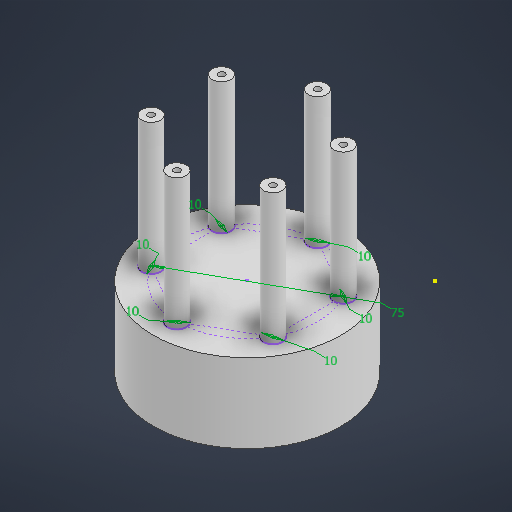
# Autodesk Inventor part: Pieza1
Saved by Autodesk Inventor 2026.1 (Build 301233000, 233)
## iProperties
Created: 2025-09-15
Part Number: Pieza1
Material: Genérico
Document SubType Name: Modeling
Designer: Usuario
Density: 1 g/cm^3
Appearance: Valor por defecto
Author: Usuario
Autodesk Inventor part; units mm, degrees
ref_plane "YZ Plane" through (0, 0, 0) normal (1, 0, 0) x (0, 1, 0)
ref_plane "XZ Plane" through (0, 0, 0) normal (0, 1, 0) x (-1, 0, 0)
ref_plane "XY Plane" through (0, 0, 0) normal (0, 0, 1) x (1, 0, 0)
sketch "Boceto1" plane through (0, 0, 0) normal (0, 1, 0) x (-1, 0, 0)
  line L0 (0, 0) -> (100, 0) construction
  line L1 (100, 0) -> (100, 100) construction
  line L2 (100, 100) -> (0, 100) construction
  line L3 (0, 100) -> (0, 0) construction
  line L4 (0, 100) -> (100, 0) construction
  line L5 (100, 100) -> (0, 0) construction
  circle A0 centre (50, 50) radius 50
  dimension "d2" = 100
  constraints: 12 end point, 2 parallel, 1 centre point, 1 horizontal, 1 midpoint, 1 perpendicular
  measures "d2" diameter of A0
extrude "Extrusión1" add sketch "Boceto1" along normal blind 35
sketch "Boceto2" plane through (-50, 35, 50) normal (0, 1, 0) x (1, 0, 0)
  circle A0 centre (0, 0) radius 37.5 construction
  line L0 (0, 37.5) -> (32.476, 18.75) construction
  line L1 (32.476, 18.75) -> (32.476, -18.75) construction
  line L2 (32.476, -18.75) -> (0, -37.5) construction
  line L3 (0, -37.5) -> (-32.476, -18.75) construction
  line L4 (-32.476, -18.75) -> (-32.476, 18.75) construction
  line L5 (-32.476, 18.75) -> (0, 37.5) construction
  circle A1 centre (0, 37.5) radius 5
  circle A2 centre (32.476, 18.75) radius 5
  circle A3 centre (32.476, -18.75) radius 5
  circle A4 centre (0, -37.5) radius 5
  circle A5 centre (-32.476, -18.75) radius 5
  circle A6 centre (-32.476, 18.75) radius 5
  point P0 (50, 50)
  dimension "d5" = 75
  dimension "d6" = 10
  dimension "d7" = 10
  dimension "d8" = 10
  dimension "d9" = 10
  dimension "d10" = 10
  dimension "d11" = 10
  constraints: 12 end point, 7 coincident, 6 centre point, 1 vertical alignment, 15 other
  measures "d6" diameter of A1
  measures "d7" diameter of A2
  measures "d8" diameter of A3
  measures "d9" diameter of A4
  measures "d10" diameter of A5
  measures "d11" diameter of A6
extrude "Extrusión2" add sketch "Boceto2" along normal blind 70
sketch "Boceto3" plane through (-82.476, 105, 68.75) normal (0, 1, 0) x (1, 0, 0)
  circle A0 centre (32.5355, 18.7491) radius 37.5 construction
  circle A1 centre (32.5355, -18.7509) radius 1.75
  circle A2 centre (65.012, 0) radius 1.75
  circle A3 centre (65.012, 37.4981) radius 1.75
  circle A4 centre (32.5355, 56.2491) radius 1.75
  circle A5 centre (0.059, 37.4981) radius 1.75
  circle A6 centre (0, 0) radius 5 projected
  circle A7 centre (0, 0) radius 1.75
  point P0 (82.476, 68.75)
  dimension "d15" = 3.5
  dimension "d16" = 3.5
  dimension "d17" = 3.5
  dimension "d18" = 3.5
  dimension "d19" = 3.5
  dimension "d20" = 3.5
  constraints: 7 centre point, 5 point on circle, 1 coincident
  measures "d15" diameter of A1
  measures "d16" diameter of A2
  measures "d17" diameter of A3
  measures "d18" diameter of A4
  measures "d19" diameter of A5
  measures "d20" diameter of A7
extrude "Extrusión3" cut sketch "Boceto3" against normal blind 9 contours A1 | A2 | A3 | A4 | A5 | A7
sketch "Boceto4" plane through (-50, 0, 50) normal (0, -1, 0) x (1, 0, 0)
  circle A0 centre (0, 0) radius 40
  circle A1 centre (0, 0) radius 6
  line L0 (-20, -34.641) -> (-3.5, -6.0622)
  line L1 (-20.7581, -33.3279) -> (-4.5751, -5.298)
  line L2 (20, -34.641) -> (3.5, -6.0622)
  line L3 (-18.2769, 34.641) -> (-2.199, 6.6456)
  line L4 (4.6319, -5.2484) -> (20.7581, -33.3279)
  line L5 (39.0497, -1.6459) -> (6.8037, -1.6459)
  line L6 (7, 0) -> (40, 0)
  line L7 (3.5, 6.0622) -> (20, 34.641)
  line L8 (2.3007, 6.6111) -> (18.4837, 34.641)
  arc A2 (2.3007, 6.6111) -> (-2.199, 6.6456) centre (0, 0) ccw
  arc A3 (-3.5, 6.0622) -> (-7, 0) centre (0, 0) ccw
  line L9 (-6.8037, -1.6459) -> (-39.0497, -1.6459)
  arc A4 (-6.8037, -1.6459) -> (-4.5751, -5.298) centre (0, 0) ccw
  line L10 (-40, 0) -> (-7, 0)
  arc A5 (-3.5, -6.0622) -> (3.5, -6.0622) centre (0, 0) ccw
  arc A6 (4.6319, -5.2484) -> (6.8037, -1.6459) centre (0, 0) ccw
  arc A7 (7, 0) -> (3.5, 6.0622) centre (0, 0) ccw
  line L11 (-3.5, 6.0622) -> (-20, 34.641)
  line L12 (20.7581, -33.3279) -> (21.125, -33.9667)
  line L13 (39.0497, -1.6459) -> (39.9661, -1.6459)
  line L14 (18.4837, 34.641) -> (18.852, 35.2789)
  line L15 (-18.6921, 35.3639) -> (-18.2769, 34.641)
  line L16 (-39.0497, -1.6459) -> (-39.9661, -1.6459)
  line L17 (-20.7581, -33.3279) -> (-21.125, -33.9667)
  point P0 (50, -50)
  point P1 (-20, -34.641)
  point P2 (20, 34.641)
  point P3 (-20, 34.641)
  dimension "d23" = 80
  dimension "d24" = 12
  constraints: 36 end point, 12 point on circle, 9 parallel, 7 centre point, 3 coincident, 3 horizontal, 16 other
  measures "d24" diameter of A1
extrude "Extrusión4" cut sketch "Boceto4" against normal blind 30 contours L6 A7 L7 A0 | A0 L12 L4 A6 L5 L13 | L14 L8 A2 L3 L15 A0 | A0 L0 A5 L2 | L11 A3 L10 A0 | A0 L16 L9 A4 L1 L17 | A1
sketch "Boceto5" plane through (-50, 0, 50) normal (0, -1, 0) x (1, 0, 0)
  arc A0 (-3.5, 6.0622) -> (-7, 0) centre (0, 0) ccw projected
  circle A1 centre (0, 0) radius 50
  circle A2 centre (0, 0) radius 40
  point P0 (50, -50)
  dimension "d28" = 100
  dimension "d29" = 80
  constraints: 2 centre point, 2 coincident
  measures "d28" diameter of A1
  measures "d29" diameter of A2
extrude "Extrusión5" add sketch "Boceto5" along normal blind 7
thread "Rosca1" size "M80x1.5" class "6H" standard "ANSI Metric M Profile" length 6
